Autodesk Fusion 360 part; units mm, degrees
(part 10 of 11)
  measures "d146" distance of A0.centre L904
  measures "d147" diameter of A29
  measures "d148" distance of A21.centre L241
  measures "d149" distance of A21.centre L1147
  measures "d150" diameter of A17
  measures "d151" distance of A17.centre L2172
  measures "d152" distance of A17.centre L1106
  measures "d153" diameter of A69
  measures "d154" diameter of A50
  measures "d155" diameter of A63
  measures "d156" diameter of A15
  measures "d157" diameter of A47
  measures "d158" diameter of A5
  measures "d159" distance of A5.centre L1493
  measures "d160" distance of A43.centre L926
  measures "d161" distance of A15.centre L926
  measures "d162" distance of A60.centre L796
  measures "d163" distance of A68.centre L4112
  measures "d164" distance of A17.centre L1102
  measures "d165" distance of A68.centre L4388
  measures "d166" distance of A68.centre L4363
  measures "d167" distance of A49.centre L3076
  measures "d168" distance of A49.centre L3488
  measures "d169" distance of A60.centre L3636
  measures "d170" distance of A60.centre L3768
  measures "d171" distance of A15.centre L1414
  measures "d172" distance of A15.centre L1372
  measures "d173" distance of A43.centre L577
  measures "d174" distance of A43.centre L2522
  measures "d175" distance of A5.centre L729
  measures "d176" distance of A5.centre L761
  measures "d177" distance of A17.centre L1070
  measures "d178" distance of A17.centre L1079
  measures "d179" distance of A21.centre L1134
  measures "d180" distance of A21.centre L1105
  measures "d181" distance of A0.centre L205
  measures "d182" distance of A0.centre L871
  measures "d183" distance of A53.centre L2428
  measures "d184" distance of A53.centre L3199
  measures "d185" distance of A39.centre L4631
  measures "d186" distance of A39.centre L1477
  measures "d187" distance of A36.centre L1441
  measures "d188" radius of A32
  measures "d189" distance of L2406 L2562
  measures "d190" distance of L2398 L2487
  measures "d191" distance of L2399 L2562
  measures "d192" distance of L2398 L2532
  measures "d193" distance of L2406 L2546
  measures "d194" distance of L2487 L2580
  measures "d195" distance of L2490 L2532
  measures "d196" distance of L1493 L2399
sketch "Sketch3" plane through (0, 0, 0) normal (0, 0, 1) x (1, 0, 0)
  line L0 (-169.0689, -23.2426) -> (259.656, -23.2426)
  arc A0 (-174.0689, -18.2426) -> (-169.0689, -23.2426) centre (-169.0689, -18.2426) ccw
  line L1 (-174.0689, 118.4832) -> (-174.0689, -18.2426)
  arc A1 (-169.0689, 123.4832) -> (-174.0689, 118.4832) centre (-169.0689, 118.4832) ccw
  line L2 (-158.7961, 123.4832) -> (-169.0689, 123.4832)
  line L3 (259.656, 123.4832) -> (-158.7961, 123.4832)
  arc A2 (264.656, 118.4832) -> (259.656, 123.4832) centre (259.656, 118.4832) ccw
  line L4 (264.656, -18.2426) -> (264.656, 118.4832)
  arc A3 (259.656, -23.2426) -> (264.656, -18.2426) centre (259.656, -18.2426) ccw
  line L5 (260.257, 83.109) -> (260.257, -11.1417)
  line L6 (257.232, 0.4083) -> (257.232, 14.4091)
  line L7 (209.607, -9.1167) -> (195.605, -9.1167)
  line L8 (162.267, 109.6602) -> (176.267, 109.6602)
  line L9 (-166.345, 99.7592) -> (-166.345, 105.5592)
  line L10 (205.13, 81.084) -> (219.132, 81.084)
  line L11 (143.217, 95.6582) -> (157.217, 95.6582)
  line L12 (114.998, -11.1417) -> (114.998, 83.109)
  line L13 (183.055, 83.109) -> (183.055, -11.1417)
  line L14 (-131.2701, 111.6852) -> (-131.2701, 93.6332)
  line L15 (-149.3191, 93.6332) -> (-149.3191, 111.6852)
  line L16 (-45.545, 111.6852) -> (-45.545, 93.6332)
  line L17 (-54.069, 93.6332) -> (-54.069, 111.6852)
  line L18 (40.18, 111.6852) -> (40.18, 93.6332)
  line L19 (31.656, 93.6332) -> (31.656, 111.6852)
  line L20 (121.142, 111.6852) -> (121.142, 93.6332)
  line L21 (117.381, 93.6332) -> (117.381, 111.6852)
  line L22 (179.292, 93.6332) -> (179.292, 111.6852)
  line L23 (185.808, 109.3822) -> (198.508, 109.3822)
  line L24 (185.808, 96.3822) -> (185.808, 109.3822)
  line L25 (198.508, 96.3822) -> (185.808, 96.3822)
  line L26 (198.508, 109.3822) -> (198.508, 96.3822)
  line L27 (-152.3441, 99.7592) -> (-152.3441, 105.5592)
  line L28 (-128.2451, 105.5592) -> (-128.2451, 99.7592)
  line L29 (43.205, 99.7592) -> (43.205, 105.5592)
  line L30 (114.356, 105.5592) -> (114.356, 99.7592)
  line L31 (-57.094, 99.7592) -> (-57.094, 105.5592)
  line L32 (-42.52, 99.7592) -> (-42.52, 105.5592)
  line L33 (28.631, 105.5592) -> (28.631, 99.7592)
  line L34 (124.167, 105.5592) -> (124.167, 99.7592)
  line L35 (176.267, 105.5592) -> (176.267, 99.7592)
  line L36 (186.08, 52.1344) -> (186.08, 57.9344)
  line L37 (176.267, 57.9344) -> (176.267, 52.1344)
  line L38 (111.973, -5.0157) -> (111.973, 0.7845)
  line L39 (124.167, -5.0157) -> (124.167, 0.7845)
  line L40 (-168.37, 112.6852) -> (-150.3191, 112.6852)
  line L41 (-168.37, 92.6332) -> (-150.3191, 92.6332)
  line L42 (-130.2701, 92.6332) -> (-55.069, 92.6332)
  line L43 (-130.2701, 112.6852) -> (-55.069, 112.6852)
  line L44 (-44.545, 92.6332) -> (30.656, 92.6332)
  line L45 (-44.545, 112.6852) -> (30.656, 112.6852)
  line L46 (41.18, 92.6332) -> (116.381, 92.6332)
  line L47 (122.142, 92.6332) -> (178.292, 92.6332)
  line L48 (113.998, 84.109) -> (-168.37, 84.109)
  line L49 (41.18, 112.6852) -> (116.381, 112.6852)
  line L50 (122.142, 112.6852) -> (178.292, 112.6852)
  line L51 (259.257, 84.109) -> (184.055, 84.109)
  line L52 (178.292, 84.109) -> (122.142, 84.109)
  line L53 (259.257, -12.1417) -> (184.055, -12.1417)
  line L54 (178.292, -12.1417) -> (122.142, -12.1417)
  line L55 (113.998, -12.1417) -> (-168.37, -12.1417)
  line L56 (-169.37, -11.1417) -> (-169.37, 83.109)
  line L57 (-169.37, 93.6332) -> (-169.37, 111.6852)
  line L58 (185.808, 109.3822) -> (198.508, 96.3822)
  circle A4 centre (192.158, 102.8822) radius 3.75
  circle A5 centre (192.158, 102.8822) radius 9.25
  arc A6 (-168.37, 112.6852) -> (-169.37, 111.6852) centre (-168.37, 111.6852) ccw
  arc A7 (-169.37, 93.6332) -> (-168.37, 92.6332) centre (-168.37, 93.6332) ccw
  arc A8 (-150.3191, 92.6332) -> (-149.3191, 93.6332) centre (-150.3191, 93.6332) ccw
  arc A9 (-149.3191, 111.6852) -> (-150.3191, 112.6852) centre (-150.3191, 111.6852) ccw
  arc A10 (-130.2701, 112.6852) -> (-131.2701, 111.6852) centre (-130.2701, 111.6852) ccw
  arc A11 (-131.2701, 93.6332) -> (-130.2701, 92.6332) centre (-130.2701, 93.6332) ccw
  arc A12 (-54.069, 111.6852) -> (-55.069, 112.6852) centre (-55.069, 111.6852) ccw
  arc A13 (-55.069, 92.6332) -> (-54.069, 93.6332) centre (-55.069, 93.6332) ccw
  arc A14 (-45.545, 93.6332) -> (-44.545, 92.6332) centre (-44.545, 93.6332) ccw
  arc A15 (-44.545, 112.6852) -> (-45.545, 111.6852) centre (-44.545, 111.6852) ccw
  arc A16 (31.656, 111.6852) -> (30.656, 112.6852) centre (30.656, 111.6852) ccw
  arc A17 (30.656, 92.6332) -> (31.656, 93.6332) centre (30.656, 93.6332) ccw
  arc A18 (40.18, 93.6332) -> (41.18, 92.6332) centre (41.18, 93.6332) ccw
  arc A19 (41.18, 112.6852) -> (40.18, 111.6852) centre (41.18, 111.6852) ccw
  arc A20 (117.381, 111.6852) -> (116.381, 112.6852) centre (116.381, 111.6852) ccw
  arc A21 (116.381, 92.6332) -> (117.381, 93.6332) centre (116.381, 93.6332) ccw
  arc A22 (121.142, 93.6332) -> (122.142, 92.6332) centre (122.142, 93.6332) ccw
  arc A23 (122.142, 112.6852) -> (121.142, 111.6852) centre (122.142, 111.6852) ccw
  arc A24 (179.292, 111.6852) -> (178.292, 112.6852) centre (178.292, 111.6852) ccw
  arc A25 (178.292, 92.6332) -> (179.292, 93.6332) centre (178.292, 93.6332) ccw
  arc A26 (184.055, 84.109) -> (183.055, 83.109) centre (184.055, 83.109) ccw
  arc A27 (260.257, 83.109) -> (259.257, 84.109) centre (259.257, 83.109) ccw
  arc A28 (259.257, -12.1417) -> (260.257, -11.1417) centre (259.257, -11.1417) ccw
  arc A29 (183.055, -11.1417) -> (184.055, -12.1417) centre (184.055, -11.1417) ccw
  arc A30 (179.292, 83.109) -> (178.292, 84.109) centre (178.292, 83.109) ccw
  arc A31 (178.292, -12.1417) -> (179.292, -11.1417) centre (178.292, -11.1417) ccw
  arc A32 (121.142, -11.1417) -> (122.142, -12.1417) centre (122.142, -11.1417) ccw
  arc A33 (122.142, 84.109) -> (121.142, 83.109) centre (122.142, 83.109) ccw
  arc A34 (114.998, 83.109) -> (113.998, 84.109) centre (113.998, 83.109) ccw
  arc A35 (113.998, -12.1417) -> (114.998, -11.1417) centre (113.998, -11.1417) ccw
  arc A36 (-169.37, -11.1417) -> (-168.37, -12.1417) centre (-168.37, -11.1417) ccw
  arc A37 (-168.37, 84.109) -> (-169.37, 83.109) centre (-168.37, 83.109) ccw
  line L59 (-152.3441, 109.6602) -> (-166.345, 109.6602)
  line L60 (-166.345, 95.6582) -> (-152.3441, 95.6582)
  line L61 (-171.5689, 114.6832) -> (262.156, 114.6832)
  line L62 (-171.5689, 114.6832) -> (-171.5689, -14.4426)
  line L63 (262.156, -14.4426) -> (-171.5689, -14.4426)
  line L64 (262.156, 114.6832) -> (262.156, -14.4426)
  line L65 (122.142, 45.0083) -> (178.292, 45.0083)
  line L66 (124.167, 48.0333) -> (138.167, 48.0333)
  line L67 (141.192, 26.959) -> (159.242, 26.959)
  line L68 (143.217, 23.934) -> (157.217, 23.934)
  line L69 (140.192, 25.959) -> (140.192, 8.9091)
  line L70 (160.242, 25.959) -> (160.242, 26)
  line L71 (160.242, 26) -> (160.242, 8.9091)
  line L72 (143.217, 19.8345) -> (143.217, 14.0343)
  line L73 (157.217, 19.8345) -> (157.217, 14.0343)
  line L74 (122.142, 7.9091) -> (139.192, 7.9091)
  line L75 (161.242, 7.9091) -> (178.292, 7.9091)
  line L76 (162.267, 4.8841) -> (176.267, 4.8841)
  line L77 (124.167, 4.8841) -> (138.167, 4.8841)
  line L78 (121.142, 83.109) -> (121.142, 46.0083)
  line L79 (121.142, 6.9091) -> (121.142, -11.1417)
  line L80 (179.292, -11.1417) -> (179.292, 6.9091)
  line L81 (179.292, 46.0083) -> (179.292, 83.109)
  arc A38 (121.142, 46.0083) -> (122.142, 45.0083) centre (122.142, 46.0083) ccw
  arc A39 (178.292, 45.0083) -> (179.292, 46.0083) centre (178.292, 46.0083) ccw
  arc A40 (160.242, 25.959) -> (159.242, 26.959) centre (159.242, 25.959) ccw
  arc A41 (141.192, 26.959) -> (140.192, 25.959) centre (141.192, 25.959) ccw
  arc A42 (122.142, 7.9091) -> (121.142, 6.9091) centre (122.142, 6.9091) ccw
  arc A43 (179.292, 6.9091) -> (178.292, 7.9091) centre (178.292, 6.9091) ccw
  arc A44 (139.192, 7.9091) -> (140.192, 8.9091) centre (139.192, 8.9091) ccw
  arc A45 (160.242, 8.9091) -> (161.242, 7.9091) centre (161.242, 8.9091) ccw
  dimension "d197" = 3.025
  dimension "d198" = 3.025
  dimension "d199" = 3.025
  dimension "d200" = 3.025
  dimension "d201" = 3.025
  dimension "d202" = 3.025
  dimension "d203" = 3.025
  dimension "d204" = 3.025
  dimension "d205" = 3.025
  dimension "d206" = 3.025
  dimension "d207" = 3.025
  dimension "d208" = 3.025
  dimension "d209" = 3.025
  dimension "d210" = 3.025
  dimension "d211" = 3.025
  dimension "d212" = 3.025
  dimension "d213" = 3.025
  dimension "d214" = 3.025
  dimension "d215" = 3.025
  dimension "d216" = 7.5
  dimension "d218" = 18.5
  dimension "d219" = 1
  dimension "d240" = 3.025
  dimension "d241" = 3.025
  dimension "d242" = 3.025
  dimension "d243" = 3.025
  dimension "d244" = 3.025
  dimension "d245" = 3.025
  dimension "d246" = 1
  dimension "d247" = 1
  constraint horizontal L40
  constraint vertical L5
  constraint horizontal L53
  constraint vertical L56
  constraint horizontal L41
  constraint horizontal L51
  constraint vertical L78
  constraint vertical L12
  constraint vertical L13
  constraint vertical L80
  constraint vertical L14
  constraint vertical L15
  constraint vertical L16
  constraint vertical L17
  constraint vertical L18
  constraint vertical L19
  constraint vertical L20
  constraint vertical L21
  constraint vertical L22
  constraint collinear L40 L43
  constraint collinear L41 L42
  constraint collinear L42 L44
  constraint collinear L43 L45
  constraint collinear L44 L46
  constraint collinear L45 L49
  constraint collinear L46 L47
  constraint collinear L48 L52
  constraint collinear L49 L50
  constraint collinear L51 L52
  constraint collinear L53 L54
  constraint collinear L54 L55
  constraint collinear L56 L57
  constraint coincident L23.start L24.end
  constraint coincident L25.start L26.end
  constraint midpoint L58 A4.centre
  constraint tangent L40 A6
  constraint tangent L57 A6
  constraint tangent L41 A7
  constraint tangent L57 A7
  constraint equal A6 A7
  constraint tangent L15 A8
  constraint tangent L41 A8
  constraint equal A6 A8
  constraint tangent L15 A9
  constraint tangent L40 A9
  constraint equal A6 A9
  constraint tangent L14 A10
  constraint tangent L43 A10
  constraint equal A6 A10
  constraint tangent L14 A11
  constraint tangent L42 A11
  constraint equal A6 A11
  constraint tangent L17 A12
  constraint tangent L43 A12
  constraint equal A6 A12
  constraint tangent L17 A13
  constraint tangent L42 A13
  constraint equal A6 A13
  constraint tangent L16 A14
  constraint tangent L44 A14
  constraint equal A6 A14
  constraint tangent L16 A15
  constraint tangent L45 A15
  constraint equal A6 A15
  constraint tangent L19 A16
  constraint tangent L45 A16
  constraint equal A6 A16
  constraint tangent L19 A17
  constraint tangent L44 A17
  constraint equal A6 A17
  constraint tangent L18 A18
  constraint tangent L46 A18
  constraint equal A6 A18
  constraint tangent L18 A19
  constraint tangent L49 A19
  constraint equal A6 A19
  constraint tangent L21 A20
  constraint tangent L49 A20
  constraint equal A6 A20
  constraint tangent L21 A21
  constraint tangent L46 A21
  constraint equal A6 A21
  constraint tangent L20 A22
  constraint tangent L47 A22
  constraint equal A6 A22
  constraint tangent L20 A23
  constraint tangent L50 A23
  constraint equal A6 A23
  constraint tangent L50 A24
  constraint tangent L22 A24
  constraint equal A6 A24
  constraint tangent L47 A25
  constraint tangent L22 A25
  constraint equal A6 A25
  constraint tangent L51 A26
  constraint tangent L13 A26
  constraint equal A6 A26
  constraint tangent L51 A27
  constraint tangent L5 A27
  constraint equal A6 A27
  constraint tangent L5 A28
  constraint tangent L53 A28
  constraint equal A6 A28
  constraint tangent L53 A29
  constraint tangent L13 A29
  constraint equal A6 A29
  constraint tangent A30 L81
  constraint tangent L52 A30
  constraint equal A6 A30
  constraint tangent A31 L80
  constraint tangent L54 A31
  constraint equal A6 A31
  constraint tangent L54 A32
  constraint tangent A32 L79
  constraint equal A6 A32
  constraint tangent A33 L78
  constraint tangent L52 A33
  constraint equal A6 A33
  constraint tangent L48 A34
  constraint tangent L12 A34
  constraint equal A6 A34
  constraint tangent L55 A35
  constraint tangent L12 A35
  constraint equal A6 A35
  constraint tangent L55 A36
  constraint tangent L56 A36
  constraint equal A6 A36
  constraint tangent L56 A37
  constraint tangent L48 A37
  constraint equal A6 A37
  constraint perpendicular L65 L81
  constraint perpendicular L67 L81
  constraint perpendicular L67 L69
  constraint perpendicular L67 L70
  constraint parallel L70 L71
  constraint perpendicular L69 L74
  constraint perpendicular L75 L80
  constraint collinear L78 L79
  constraint collinear L80 L81
  constraint tangent L65 A38
  constraint tangent L78 A38
  constraint tangent L65 A39
  constraint tangent L81 A39
  constraint equal A38 A39
  constraint tangent L70 A40
  constraint tangent L67 A40
  constraint equal A38 A40
  constraint tangent L69 A41
  constraint tangent L67 A41
  constraint equal A38 A41
  constraint tangent L74 A42
  constraint tangent L79 A42
  constraint equal A38 A42
  constraint tangent L75 A43
  constraint tangent L80 A43
  constraint equal A38 A43
  constraint tangent L74 A44
  constraint tangent L69 A44
  constraint tangent L75 A45
  constraint tangent L71 A45
  constraint equal A44 A45
  measures "d197" distance of L5 L6
  measures "d198" distance of L7 L53
  measures "d199" distance of L8 L50
  measures "d200" distance of L9 L57
  measures "d201" distance of L10 L51
  measures "d202" distance of L11 L47
  measures "d203" distance of L15 L27
  measures "d204" distance of L14 L28
  measures "d205" distance of L18 L29
  measures "d206" distance of L21 L30
  measures "d207" distance of L17 L31
  measures "d208" distance of L16 L32
  measures "d209" distance of L19 L33
  measures "d210" distance of L20 L34
  measures "d211" distance of L22 L35
  measures "d212" distance of L13 L36
  measures "d213" distance of L37 L81
  measures "d214" distance of L12 L38
  measures "d215" distance of L39 L79
  measures "d216" diameter of A4
  measures "d218" diameter of A5
  measures "d219" radius of A6
  measures "d240" distance of L65 L66
  measures "d241" distance of L67 L68
  measures "d242" distance of L69 L72
  measures "d243" distance of L71 L73
  measures "d244" distance of L75 L76
  measures "d245" distance of L74 L77
  measures "d246" radius of A38
  measures "d247" radius of A44
extrude "Extrude2" add sketch "Sketch1" along normal blind 4.5 contours A12 A13 L19 L32 L42 L48 A44 A52 L78 L89 makes body 1
extrude "Extrude3" add sketch "Sketch1" along normal blind 3 from surface at 4.5 separate body contours L0 L2 L4 A5 A7 A28 A35 L90 A97 L124 L125 | A1 L5 A10 L16 A19 A22 L65 L90 L122 A96 L123 | L90 A97 L124 L125 | L90 L122 A96 L123 | L49 A42 A43 L54 A55 L67 A57 L90 L120 A95 L121 | L90 L120 A95 L121 | A4 A11 L10 L12 A14 A18 L33 L95 L102 L103 A86 | L95 L102 L103 A86 | L72 L73 A62 A64 A67 L84 A71 L90 L118 A94 L119 | L90 L118 A94 L119 | A21 A24 L25 L26 A34 A36 L36 L95 L104 A87 L105 | L95 L104 A87 L105 | L37 A41 A46 L59 A51 L63 A59 L90 A93 L116 L117 | L90 A93 L116 L117 | L22 L27 A27 A29 L29 A31 A32 L95 L106 A88 L107 | L95 L106 A88 L107 | L41 L43 A40 A49 A50 L64 A58 L90 L114 A92 L115 | L90 L114 A92 L115 | L74 L75 A63 L77 A65 A68 A69 L95 L108 A89 L109 | L95 L108 A89 L109 | A75 L93 L95 A81 A82 L99 L100 A85 L110 A90 L111 | L57 A73 L87 L88 A76 A77 L95 A80 L112 A91 L113 | L95 L110 A90 L111 | L95 L112 A91 L113 | A0 | A2 | A3 | A6 | A8 | A9 | A12 A13 L19 L32 L42 L48 A44 A52 L78 L89 | A15 | A16 | A17 | A20 | A23 | A25 | A26 | A30 | A33 | A37 | A38 | A39 | A45 | A47 | A48 | A53 | A54 | A56 | A60 | A61 | A66 | A70 | A72 | A74 | A78 | A79 | A83 | A84 | A98 | A99 makes body 2
extrude "Extrude4" add sketch "Sketch3" along normal blind 6 from surface at 1.5 separate body contours L61 L62 L63 L64 makes body 3
combine "Combine1" operation add target body 3 tool bodies 2 1
extrude "Extrude5" add sketch "Sketch3" along normal blind 3 from surface at 1.5 contours L24 L25 L58 A4 | L23 L26 L58 A4 | A5 bodies 3
sketch "Sketch4" plane through (0, 0, 0) normal (0, 0, 1) x (1, 0, 0)
  spline S0 degree 3 poles (218.2871, 110.1253) (218.4274, 110.1253) (218.5464, 110.0777) (218.6417, 109.9811) knots 0 0 0 0 1 1 1 1
  spline S1 degree 3 poles (218.6417, 109.9811) (218.7369, 109.8859) (218.7859, 109.7734) (218.7859, 109.6451) knots 0 0 0 0 1 1 1 1
  line L0 (218.7859, 109.6451) -> (218.7859, 107.4993)
  spline S2 degree 3 poles (218.7859, 107.4993) (218.7859, 107.3591) (218.7382, 107.244) (218.6417, 107.154) knots 0 0 0 0 1 1 1 1
  spline S3 degree 3 poles (218.6417, 107.154) (218.5464, 107.0641) (218.4274, 107.0204) (218.2871, 107.0204) knots 0 0 0 0 1 1 1 1
  line L1 (218.2871, 107.0204) -> (213.8408, 107.0204)
  spline S4 degree 3 poles (213.8408, 107.0204) (214.1213, 107.0204) (214.3739, 106.9186) (214.5975, 106.7135) knots 0 0 0 0 1 1 1 1
  spline S5 degree 3 poles (214.5975, 106.7135) (214.8211, 106.5084) (214.9335, 106.2796) (214.9335, 106.0243) knots 0 0 0 0 1 1 1 1
  line L2 (214.9335, 106.0243) -> (214.9335, 97.2467)
  spline S6 degree 3 poles (214.9335, 97.2467) (214.9335, 97.1065) (214.8819, 96.998) (214.7801, 96.9213) knots 0 0 0 0 1 1 1 1
  spline S7 degree 3 poles (214.7801, 96.9213) (214.6901, 96.8313) (214.575, 96.7877) (214.4348, 96.7877) knots 0 0 0 0 1 1 1 1
  line L3 (214.4348, 96.7877) -> (211.7704, 96.7877)
  spline S8 degree 3 poles (211.7704, 96.7877) (211.6302, 96.7877) (211.5151, 96.8326) (211.4252, 96.9213) knots 0 0 0 0 1 1 1 1
  spline S9 degree 3 poles (211.4252, 96.9213) (211.3233, 96.998) (211.2717, 97.1065) (211.2717, 97.2467) knots 0 0 0 0 1 1 1 1
  line L4 (211.2717, 97.2467) -> (211.2717, 106.4463)
  spline S10 degree 3 poles (211.2717, 106.4463) (211.2717, 106.6249) (211.2148, 106.7651) (211.0997, 106.8683) knots 0 0 0 0 1 1 1 1
  spline S11 degree 3 poles (211.0997, 106.8683) (210.9846, 106.9701) (210.851, 107.0217) (210.6976, 107.0217) knots 0 0 0 0 1 1 1 1
  line L5 (210.6976, 107.0217) -> (207.9194, 107.0217)
  spline S12 degree 3 poles (207.9194, 107.0217) (207.7911, 107.0217) (207.676, 107.0667) (207.5741, 107.1554) knots 0 0 0 0 1 1 1 1
  spline S13 degree 3 poles (207.5741, 107.1554) (207.4723, 107.244) (207.4207, 107.3591) (207.4207, 107.5006) knots 0 0 0 0 1 1 1 1
  line L6 (207.4207, 107.5006) -> (207.4207, 108.4783)
  spline S14 degree 3 poles (207.4207, 108.4783) (207.4207, 108.7204) (207.4683, 108.9439) (207.5649, 109.149) knots 0 0 0 0 1 1 1 1
  spline S15 degree 3 poles (207.5649, 109.149) (207.6601, 109.3527) (207.7885, 109.5287) (207.9485, 109.6755) knots 0 0 0 0 1 1 1 1
  spline S16 degree 3 poles (207.9485, 109.6755) (208.1086, 109.8224) (208.2872, 109.9348) (208.4856, 110.0115) knots 0 0 0 0 1 1 1 1
  spline S17 degree 3 poles (208.4856, 110.0115) (208.6841, 110.0883) (208.8852, 110.1266) (209.0889, 110.1266) knots 0 0 0 0 1 1 1 1
  line L7 (209.0889, 110.1266) -> (218.2871, 110.1266)
  line L8 (218.2871, 110.1266) -> (218.2871, 110.1253)
  line L9 (220.4911, 97.2282) -> (220.4911, 108.4386)
  spline S18 degree 3 poles (220.4911, 108.4386) (220.4911, 108.9241) (220.6565, 109.3236) (220.9898, 109.6358) knots 0 0 0 0 1 1 1 1
  spline S19 degree 3 poles (220.9898, 109.6358) (221.3219, 109.9494) (221.7122, 110.1055) (222.1593, 110.1055) knots 0 0 0 0 1 1 1 1
  line L10 (222.1593, 110.1055) -> (229.9777, 110.1055)
  spline S20 degree 3 poles (229.9777, 110.1055) (230.118, 110.1055) (230.237, 110.0578) (230.3323, 109.9613) knots 0 0 0 0 1 1 1 1
  spline S21 degree 3 poles (230.3323, 109.9613) (230.4275, 109.866) (230.4765, 109.7469) (230.4765, 109.6067) knots 0 0 0 0 1 1 1 1
  line L11 (230.4765, 109.6067) -> (230.4765, 107.7097)
  spline S22 degree 3 poles (230.4765, 107.7097) (230.4765, 107.5694) (230.4315, 107.4609) (230.3429, 107.3842) knots 0 0 0 0 1 1 1 1
  spline S23 degree 3 poles (230.3429, 107.3842) (230.2529, 107.2943) (230.1325, 107.2506) (229.9791, 107.2506) knots 0 0 0 0 1 1 1 1
  line L12 (229.9791, 107.2506) -> (222.9081, 107.2506)
  spline S24 degree 3 poles (222.9081, 107.2506) (223.215, 107.2506) (223.4663, 107.1421) (223.6648, 106.9252) knots 0 0 0 0 1 1 1 1
  spline S25 degree 3 poles (223.6648, 106.9252) (223.8632, 106.7082) (223.9624, 106.4714) (223.9624, 106.2161) knots 0 0 0 0 1 1 1 1
  line L13 (223.9624, 106.2161) -> (223.9624, 105.4117)
  spline S26 degree 3 poles (223.9624, 105.4117) (223.9624, 105.2715) (224.0101, 105.1366) (224.1066, 105.0096) knots 0 0 0 0 1 1 1 1
  spline S27 degree 3 poles (224.1066, 105.0096) (224.2019, 104.8813) (224.3461, 104.8178) (224.5379, 104.8178) knots 0 0 0 0 1 1 1 1
  line L14 (224.5379, 104.8178) -> (228.7157, 104.8178)
  spline S28 degree 3 poles (228.7157, 104.8178) (228.8559, 104.8178) (228.975, 104.7701) (229.0702, 104.6736) knots 0 0 0 0 1 1 1 1
  spline S29 degree 3 poles (229.0702, 104.6736) (229.1655, 104.5783) (229.2144, 104.4592) (229.2144, 104.319) knots 0 0 0 0 1 1 1 1
  line L15 (229.2144, 104.319) -> (229.2144, 102.5939)
  spline S30 degree 3 poles (229.2144, 102.5939) (229.2144, 102.4537) (229.1668, 102.3346) (229.0702, 102.2394) knots 0 0 0 0 1 1 1 1
  spline S31 degree 3 poles (229.0702, 102.2394) (228.975, 102.1441) (228.8559, 102.0952) (228.7157, 102.0952) knots 0 0 0 0 1 1 1 1
  line L16 (228.7157, 102.0952) -> (222.9094, 102.0952)
  spline S32 degree 3 poles (222.9094, 102.0952) (223.2031, 102.0952) (223.4518, 101.9933) (223.6568, 101.7883) knots 0 0 0 0 1 1 1 1
  spline S33 degree 3 poles (223.6568, 101.7883) (223.8606, 101.5832) (223.9638, 101.3544) (223.9638, 101.099) knots 0 0 0 0 1 1 1 1
  line L17 (223.9638, 101.099) -> (223.9638, 100.1981)
  spline S34 degree 3 poles (223.9638, 100.1981) (223.9638, 100.0579) (224.014, 99.923) (224.1172, 99.796) knots 0 0 0 0 1 1 1 1
  spline S35 degree 3 poles (224.1172, 99.796) (224.2191, 99.6676) (224.3593, 99.6041) (224.5392, 99.6041) knots 0 0 0 0 1 1 1 1
  line L18 (224.5392, 99.6041) -> (230.1352, 99.6041)
  spline S36 degree 3 poles (230.1352, 99.6041) (230.4672, 99.6041) (230.6339, 99.4375) (230.6339, 99.1054) knots 0 0 0 0 1 1 1 1
  line L19 (230.6339, 99.1054) -> (230.6339, 97.2269)
  spline S37 degree 3 poles (230.6339, 97.2269) (230.6339, 97.0734) (230.5863, 96.9557) (230.4897, 96.8723) knots 0 0 0 0 1 1 1 1
  spline S38 degree 3 poles (230.4897, 96.8723) (230.3945, 96.789) (230.2754, 96.748) (230.1352, 96.748) knots 0 0 0 0 1 1 1 1
  line L20 (230.1352, 96.748) -> (220.9753, 96.748)
  spline S39 degree 3 poles (220.9753, 96.748) (220.847, 96.748) (220.7358, 96.7956) (220.6406, 96.8922) knots 0 0 0 0 1 1 1 1
  spline S40 degree 3 poles (220.6406, 96.8922) (220.5453, 96.9874) (220.4964, 97.0999) (220.4964, 97.2282) knots 0 0 0 0 1 1 1 1
  line L21 (220.4964, 97.2282) -> (220.4911, 97.2282)
  line L22 (232.7757, 97.1898) -> (232.7757, 108.4002)
  spline S41 degree 3 poles (232.7757, 108.4002) (232.7757, 108.8857) (232.945, 109.2853) (233.2837, 109.5975) knots 0 0 0 0 1 1 1 1
  spline S42 degree 3 poles (233.2837, 109.5975) (233.6224, 109.911) (234.0087, 110.0671) (234.4426, 110.0671) knots 0 0 0 0 1 1 1 1
  line L23 (234.4426, 110.0671) -> (238.2751, 110.0671)
  spline S43 degree 3 poles (238.2751, 110.0671) (239.131, 110.0671) (239.9195, 109.9679) (240.6418, 109.7694) knots 0 0 0 0 1 1 1 1
  spline S44 degree 3 poles (240.6418, 109.7694) (241.3641, 109.571) (241.9925, 109.2588) (242.5296, 108.8302) knots 0 0 0 0 1 1 1 1
  spline S45 degree 3 poles (242.5296, 108.8302) (243.0667, 108.4015) (243.4874, 107.8591) (243.7943, 107.2017) knots 0 0 0 0 1 1 1 1
  spline S46 degree 3 poles (243.7943, 107.2017) (244.1012, 106.5428) (244.2666, 105.761) (244.293, 104.8535) knots 0 0 0 0 1 1 1 1
  spline S47 degree 3 poles (244.293, 104.8535) (244.3062, 104.6749) (244.3129, 104.4606) (244.3129, 104.2119) knots 0 0 0 0 1 1 1 1
  line L24 (244.3129, 104.2119) -> (244.3129, 102.5728)
  spline S48 degree 3 poles (244.3129, 102.5728) (244.3129, 102.3294) (244.3062, 102.119) (244.293, 101.9404) knots 0 0 0 0 1 1 1 1
  spline S49 degree 3 poles (244.293, 101.9404) (244.1779, 98.4519) (242.2041, 96.7083) (238.3716, 96.7083) knots 0 0 0 0 1 1 1 1
  line L25 (238.3716, 96.7083) -> (233.2546, 96.7083)
  spline S50 degree 3 poles (233.2546, 96.7083) (233.1144, 96.7083) (232.9993, 96.7533) (232.9093, 96.8419) knots 0 0 0 0 1 1 1 1
  spline S51 degree 3 poles (232.9093, 96.8419) (232.8194, 96.9305) (232.7757, 97.0456) (232.7757, 97.1872) knots 0 0 0 0 1 1 1 1
  line L26 (232.7757, 97.1872) -> (232.7757, 97.1898)
  spline S52 degree 3 poles (238.2751, 99.5658) (239.1059, 99.5658) (239.7051, 99.7669) (240.0769, 100.169) knots 0 0 0 0 1 1 1 1
  spline S53 degree 3 poles (240.0769, 100.169) (240.4473, 100.5712) (240.6391, 101.1744) (240.6524, 101.9801) knots 0 0 0 0 1 1 1 1
  spline S54 degree 3 poles (240.6524, 101.9801) (240.6656, 102.1587) (240.6748, 102.3664) (240.6815, 102.6032) knots 0 0 0 0 1 1 1 1
  spline S55 degree 3 poles (240.6815, 102.6032) (240.6881, 102.84) (240.6907, 103.1046) (240.6907, 103.3983) knots 0 0 0 0 1 1 1 1
  spline S56 degree 3 poles (240.6907, 103.3983) (240.6907, 103.692) (240.6868, 103.9565) (240.6815, 104.1933) knots 0 0 0 0 1 1 1 1
  spline S57 degree 3 poles (240.6815, 104.1933) (240.6748, 104.4301) (240.6656, 104.6365) (240.6524, 104.8164) knots 0 0 0 0 1 1 1 1
  spline S58 degree 3 poles (240.6524, 104.8164) (240.614, 106.4132) (239.7898, 107.2122) (238.1798, 107.2122) knots 0 0 0 0 1 1 1 1
  line L27 (238.1798, 107.2122) -> (235.3051, 107.2122)
  spline S59 degree 3 poles (235.3051, 107.2122) (235.5988, 107.2122) (235.8475, 107.1064) (236.0526, 106.8961) knots 0 0 0 0 1 1 1 1
  spline S60 degree 3 poles (236.0526, 106.8961) (236.2563, 106.6857) (236.3595, 106.4582) (236.3595, 106.2161) knots 0 0 0 0 1 1 1 1
  line L28 (236.3595, 106.2161) -> (236.3595, 100.1598)
  spline S61 degree 3 poles (236.3595, 100.1598) (236.3595, 99.9931) (236.4137, 99.8529) (236.5222, 99.7378) knots 0 0 0 0 1 1 1 1
  spline S62 degree 3 poles (236.5222, 99.7378) (236.6307, 99.6227) (236.7749, 99.5658) (236.9535, 99.5658) knots 0 0 0 0 1 1 1 1
  line L29 (236.9535, 99.5658) -> (238.2764, 99.5658)
  line L30 (238.2764, 99.5658) -> (238.2751, 99.5658)
  spline S63 degree 3 poles (257.4388, 100.7736) (257.4388, 99.9944) (257.2563, 99.3369) (256.8925, 98.7998) knots 0 0 0 0 1 1 1 1
  spline S64 degree 3 poles (256.8925, 98.7998) (256.5287, 98.2627) (256.0657, 97.8288) (255.5034, 97.4967) knots 0 0 0 0 1 1 1 1
  spline S65 degree 3 poles (255.5034, 97.4967) (254.9412, 97.1647) (254.3154, 96.9252) (253.6249, 96.7784) knots 0 0 0 0 1 1 1 1
  spline S66 degree 3 poles (253.6249, 96.7784) (252.9343, 96.6316) (252.2636, 96.5575) (251.6127, 96.5575) knots 0 0 0 0 1 1 1 1
  spline S67 degree 3 poles (251.6127, 96.5575) (250.9618, 96.5575) (250.3387, 96.621) (249.668, 96.7493) knots 0 0 0 0 1 1 1 1
  spline S68 degree 3 poles (249.668, 96.7493) (248.9973, 96.8763) (248.3808, 97.0906) (247.8186, 97.3909) knots 0 0 0 0 1 1 1 1
  spline S69 degree 3 poles (247.8186, 97.3909) (247.2563, 97.6912) (246.7867, 98.0868) (246.4097, 98.5789) knots 0 0 0 0 1 1 1 1
  spline S70 degree 3 poles (246.4097, 98.5789) (246.0327, 99.071) (245.825, 99.6809) (245.7866, 100.4085) knots 0 0 0 0 1 1 1 1
  spline S71 degree 3 poles (245.7866, 100.4085) (245.7866, 100.5236) (245.8276, 100.6188) (245.9109, 100.6956) knots 0 0 0 0 1 1 1 1
  spline S72 degree 3 poles (245.9109, 100.6956) (245.9943, 100.7723) (246.0935, 100.8106) (246.2086, 100.8106) knots 0 0 0 0 1 1 1 1
  line L31 (246.2086, 100.8106) -> (248.7579, 100.8106)
  spline S73 degree 3 poles (248.7579, 100.8106) (248.8346, 100.8106) (248.9021, 100.804) (248.9589, 100.7908) knots 0 0 0 0 1 1 1 1
  spline S74 degree 3 poles (248.9589, 100.7908) (249.0158, 100.7776) (249.0701, 100.7591) (249.1217, 100.7339) knots 0 0 0 0 1 1 1 1
  spline S75 degree 3 poles (249.1217, 100.7339) (249.2103, 100.6823) (249.3201, 100.5937) (249.4471, 100.4654) knots 0 0 0 0 1 1 1 1
  spline S76 degree 3 poles (249.4471, 100.4654) (249.6508, 100.0566) (249.9551, 99.7788) (250.3573, 99.6319) knots 0 0 0 0 1 1 1 1
  spline S77 degree 3 poles (250.3573, 99.6319) (250.7594, 99.4851) (251.1775, 99.411) (251.6127, 99.411) knots 0 0 0 0 1 1 1 1
  spline S78 degree 3 poles (251.6127, 99.411) (251.8045, 99.411) (252.0241, 99.4242) (252.2742, 99.4494) knots 0 0 0 0 1 1 1 1
  spline S79 degree 3 poles (252.2742, 99.4494) (252.5229, 99.4745) (252.7531, 99.5287) (252.9634, 99.6121) knots 0 0 0 0 1 1 1 1
  spline S80 degree 3 poles (252.9634, 99.6121) (253.1738, 99.6954) (253.3563, 99.8158) (253.5098, 99.9759) knots 0 0 0 0 1 1 1 1
  spline S81 degree 3 poles (253.5098, 99.9759) (253.6632, 100.136) (253.74, 100.3437) (253.74, 100.599) knots 0 0 0 0 1 1 1 1
  spline S82 degree 3 poles (253.74, 100.599) (253.74, 100.9443) (253.6116, 101.193) (253.3563, 101.3464) knots 0 0 0 0 1 1 1 1
  spline S83 degree 3 poles (253.3563, 101.3464) (253.101, 101.4999) (252.8324, 101.6216) (252.552, 101.7102) knots 0 0 0 0 1 1 1 1
  spline S84 degree 3 poles (252.552, 101.7102) (252.335, 101.787) (252.0757, 101.8597) (251.7754, 101.9312) knots 0 0 0 0 1 1 1 1
  spline S85 degree 3 poles (251.7754, 101.9312) (251.4751, 102.0013) (251.1272, 102.0754) (250.7303, 102.1521) knots 0 0 0 0 1 1 1 1
  spline S86 degree 3 poles (250.7303, 102.1521) (250.143, 102.2672) (249.5741, 102.4167) (249.0251, 102.6019) knots 0 0 0 0 1 1 1 1
  spline S87 degree 3 poles (249.0251, 102.6019) (248.4761, 102.7871) (247.9866, 103.0331) (247.5593, 103.3401) knots 0 0 0 0 1 1 1 1
  spline S88 degree 3 poles (247.5593, 103.3401) (247.1307, 103.647) (246.7867, 104.0333) (246.5248, 104.4989) knots 0 0 0 0 1 1 1 1
  spline S89 degree 3 poles (246.5248, 104.4989) (246.2628, 104.9646) (246.1319, 105.5361) (246.1319, 106.2134) knots 0 0 0 0 1 1 1 1
  spline S90 degree 3 poles (246.1319, 106.2134) (246.1319, 107.0561) (246.3647, 107.7811) (246.8317, 108.3883) knots 0 0 0 0 1 1 1 1
  spline S91 degree 3 poles (246.8317, 108.3883) (247.2974, 108.9955) (247.9072, 109.4586) (248.6613, 109.7774) knots 0 0 0 0 1 1 1 1
  spline S92 degree 3 poles (248.6613, 109.7774) (249.4788, 110.1094) (250.4181, 110.2761) (251.4778, 110.2761) knots 0 0 0 0 1 1 1 1
  spline S93 degree 3 poles (251.4778, 110.2761) (251.8998, 110.2761) (252.3363, 110.2404) (252.7901, 110.1703) knots 0 0 0 0 1 1 1 1
  spline S94 degree 3 poles (252.7901, 110.1703) (253.2439, 110.1002) (253.6844, 109.9851) (254.113, 109.825) knots 0 0 0 0 1 1 1 1
  spline S95 degree 3 poles (254.113, 109.825) (254.5403, 109.6649) (254.9399, 109.4546) (255.3103, 109.1926) knots 0 0 0 0 1 1 1 1
  spline S96 degree 3 poles (255.3103, 109.1926) (255.6807, 108.9307) (255.9995, 108.6145) (256.2681, 108.2441) knots 0 0 0 0 1 1 1 1
  spline S97 degree 3 poles (256.2681, 108.2441) (256.702, 107.6819) (256.9388, 107.113) (256.9771, 106.5389) knots 0 0 0 0 1 1 1 1
  spline S98 degree 3 poles (256.9771, 106.5389) (256.9771, 106.437) (256.9361, 106.3404) (256.8528, 106.2518) knots 0 0 0 0 1 1 1 1
  spline S99 degree 3 poles (256.8528, 106.2518) (256.7694, 106.1618) (256.6768, 106.1182) (256.575, 106.1182) knots 0 0 0 0 1 1 1 1
  line L32 (256.575, 106.1182) -> (253.8921, 106.1182)
  spline S100 degree 3 poles (253.8921, 106.1182) (253.6235, 106.1182) (253.4132, 106.2333) (253.2597, 106.4635) knots 0 0 0 0 1 1 1 1
  spline S101 degree 3 poles (253.2597, 106.4635) (253.183, 106.732) (252.9846, 106.9622) (252.6658, 107.1527) knots 0 0 0 0 1 1 1 1
  spline S102 degree 3 poles (252.6658, 107.1527) (252.3205, 107.3313) (251.9249, 107.4213) (251.4778, 107.4213) knots 0 0 0 0 1 1 1 1
  spline S103 degree 3 poles (251.4778, 107.4213) (251.2859, 107.4213) (251.0915, 107.408) (250.893, 107.3829) knots 0 0 0 0 1 1 1 1
  spline S104 degree 3 poles (250.893, 107.3829) (250.6946, 107.3578) (250.5134, 107.2996) (250.3467, 107.2109) knots 0 0 0 0 1 1 1 1
  spline S105 degree 3 poles (250.3467, 107.2109) (250.18, 107.121) (250.0464, 107.0032) (249.9445, 106.8564) knots 0 0 0 0 1 1 1 1
  spline S106 degree 3 poles (249.9445, 106.8564) (249.8426, 106.7095) (249.791, 106.5217) (249.791, 106.2915) knots 0 0 0 0 1 1 1 1
  spline S107 degree 3 poles (249.791, 106.2915) (249.791, 105.933) (249.9829, 105.6459) (250.3665, 105.4289) knots 0 0 0 0 1 1 1 1
  spline S108 degree 3 poles (250.3665, 105.4289) (250.7502, 105.2239) (251.4645, 105.0136) (252.5123, 104.7966) knots 0 0 0 0 1 1 1 1
  spline S109 degree 3 poles (252.5123, 104.7966) (253.1129, 104.6815) (253.7095, 104.5439) (254.3035, 104.3852) knots 0 0 0 0 1 1 1 1
  spline S110 degree 3 poles (254.3035, 104.3852) (254.8975, 104.2251) (255.424, 103.9989) (255.8844, 103.7052) knots 0 0 0 0 1 1 1 1
  spline S111 degree 3 poles (255.8844, 103.7052) (256.3448, 103.4115) (256.7178, 103.0305) (257.0049, 102.5648) knots 0 0 0 0 1 1 1 1
  spline S112 degree 3 poles (257.0049, 102.5648) (257.292, 102.0978) (257.4362, 101.5012) (257.4362, 100.7736) knots 0 0 0 0 1 1 1 1
  line L33 (257.4362, 100.7736) -> (257.4388, 100.7736)